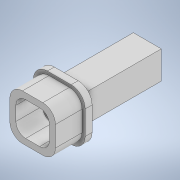
# Autodesk Inventor part: Eix Torres
Saved by Autodesk Inventor 2021 (Build 250183000, 183)
## iProperties
Created: 2021-05-03
Part Number: Eix Torres
Material: Genérico
Document SubType Name: Modeling
Designer: Marc
Density: 1 g/cm^3
Appearance: Valor por defecto
Author: Marc
## iProperties of the stored document _3DPrint.ipt
Created: 2021-05-03
Part Number: _3DPrint
Material: Genérico
Document SubType Name: Modeling
Designer: Marc
Density: 1 g/cm^3
Appearance: Valor por defecto
Author: Marc
Autodesk Inventor part; units mm, degrees
ref_plane "YZ Plane" through (0, 0, 0) normal (1, 0, 0) x (0, 1, 0)
ref_plane "XZ Plane" through (0, 0, 0) normal (0, 1, 0) x (-1, 0, 0)
ref_plane "XY Plane" through (0, 0, 0) normal (0, 0, 1) x (1, 0, 0)
sketch "Boceto1" plane through (0, 0, 0) normal (0, 0, 1) x (1, 0, 0)
  line L0 (-4.25, 9.25) -> (4.25, 9.25)
  line L1 (9.25, 4.25) -> (9.25, -4.25)
  line L2 (4.25, -9.25) -> (-4.25, -9.25)
  line L3 (-9.25, -4.25) -> (-9.25, 4.25)
  arc A0 (-4.25, 9.25) -> (-9.25, 4.25) centre (-4.25, 4.25) ccw
  arc A1 (-9.25, -4.25) -> (-4.25, -9.25) centre (-4.25, -4.25) ccw
  arc A2 (4.25, -9.25) -> (9.25, -4.25) centre (4.25, -4.25) ccw
  arc A3 (9.25, 4.25) -> (4.25, 9.25) centre (4.25, 4.25) ccw
  constraints: 8 end point, 8 point on circle, 4 centre point, 2 parallel, 1 horizontal, 1 perpendicular
extrude "Extrusión1" add sketch "Boceto1" against normal blind 2.5
sketch "Boceto3" plane through (0, 0, -2.5) normal (0, 0, -1) x (-1, 0, 0)
  line L0 (-5, -5) -> (5, -5)
  line L1 (5, -5) -> (5, 5)
  line L2 (5, 5) -> (-5, 5)
  line L3 (-5, 5) -> (-5, -5)
  constraints: 8 end point, 2 parallel, 1 horizontal, 1 perpendicular
extrude "Extrusión2" add sketch "Boceto3" along normal blind 29
sketch "Boceto4" plane through (0, 0, 0) normal (0, 0, 1) x (1, 0, 0)
  line L0 (-3.65, 8.15) -> (3.65, 8.15)
  line L1 (8.15, 3.65) -> (8.15, -3.65)
  line L2 (3.65, -8.15) -> (-3.65, -8.15)
  line L3 (-8.15, -3.65) -> (-8.15, 3.65)
  arc A0 (3.65, -8.15) -> (8.15, -3.65) centre (3.65, -3.65) ccw
  arc A1 (-8.15, -3.65) -> (-3.65, -8.15) centre (-3.65, -3.65) ccw
  arc A2 (-3.65, 8.15) -> (-8.15, 3.65) centre (-3.65, 3.65) ccw
  arc A3 (8.15, 3.65) -> (3.65, 8.15) centre (3.65, 3.65) ccw
  line L4 (-2.5, 6) -> (2.5, 6)
  line L5 (6, 2.5) -> (6, -2.5)
  line L6 (2.5, -6) -> (-2.5, -6)
  line L7 (-6, -2.5) -> (-6, 2.5)
  arc A4 (6, 2.5) -> (2.5, 6) centre (2.5, 2.5) ccw
  arc A5 (2.5, -6) -> (6, -2.5) centre (2.5, -2.5) ccw
  arc A6 (-6, -2.5) -> (-2.5, -6) centre (-2.5, -2.5) ccw
  arc A7 (-2.5, 6) -> (-6, 2.5) centre (-2.5, 2.5) ccw
  constraints: 16 end point, 16 point on circle, 8 centre point, 4 parallel, 2 horizontal, 2 perpendicular, 1 tangent
extrude "Extrusión3" add sketch "Boceto4" along normal blind 9.5
sketch "Boceto5" plane through (0, 0, -31.5) normal (0, 0, -1) x (-1, 0, 0)
  arc A0 (-1.4, 2.1909) -> (1.4, 2.1909) centre (0, 0) ccw
  line L0 (1.4, 2.1909) -> (-1.4, 2.1909)
  dimension "d36" = 5.2
  dimension "d37" = 2.8
  constraints: 2 end point, 2 point on circle, 1 centre point, 1 coincident
  measures "d36" diameter of A0
  measures "d37" distance of L0.start L0.end
extrude "Extrusión4" cut sketch "Boceto5" against normal blind 18
